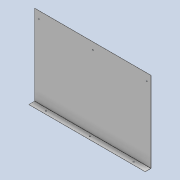
# Autodesk Inventor part: Tapa_interior_2
Saved by Autodesk Inventor 2021 (Build 250183000, 183)
## iProperties
Created: 2021-04-16
Part Number: Tapa_interior_2
Material: Genérico
Document SubType Name: Chapa
Designer: Admin
Density: 1 g/cm^3
Sheet Metal Rule: Por defecto_mm
Appearance: Valor por defecto
Flat Pattern Width: 36.1259 cm
Flat Pattern Length: 48.758 cm
Flat Pattern Area: 1761.43 cm^2
Sheet Metal Width: 361,259 mm
Sheet Metal Length: 487,580 mm
Sheet Metal Area: 176142,702 mm^2
Author: Admin
Autodesk Inventor part; units mm, degrees
ref_plane "YZ Plane" through (0, 0, 0) normal (1, 0, 0) x (0, 1, 0)
ref_plane "XZ Plane" through (0, 0, 0) normal (0, 1, 0) x (-1, 0, 0)
ref_plane "XY Plane" through (0, 0, 0) normal (0, 0, 1) x (1, 0, 0)
sketch "Boceto1" plane through (0, 0, 0) normal (0, 0, 1) x (1, 0, 0)
  line L0 (0, 0) -> (487.58, 0)
  line L1 (487.58, 0) -> (487.58, 337.58)
  line L2 (487.58, 337.58) -> (0, 337.58)
  line L3 (0, 337.58) -> (0, 0)
  dimension "d0" = 487.58
  dimension "d1" = 337.58
  measures "d0" distance of L2.end L1.end
  measures "d1" distance of L1.end L0.end
extrude "Placa1" add sketch "Boceto1" along normal blind 0.76
sketch "Boceto2" plane through (487.58, 0.76, 0) normal (0, -1, 0) x (1, 0, 0)
  line L0 (-487.58, 0) -> (0, 0)
  line L1 (0, 0) -> (0, 25)
  line L2 (0, 25) -> (-487.58, 25)
  line L3 (-487.58, 25) -> (-487.58, 0)
  constraints: 6 end point, 1 horizontal, 1 perpendicular, 1 vertical
edge flange "Pestaña1" height 25 angle 90 thickness 0.76 bend radius 0.76 thickness toward (0, -1, 0) relief straight relief width 0.76 relief depth 0.38 edges at (243.79, 0, 0.76) wall of the first edge with corners at (0, 0.76, 0) (487.58, 0.76, 0) (487.58, 0.76, 25) (0, 0.76, 25)
bend "Doblez1"
corner "Esquina1"
sketch "Boceto3" plane through (0, 0, 0) normal (0, 0, -1) x (-1, 0, 0)
  circle A0 centre (-469.48, 308.225) radius 2.5 projected
  circle A1 centre (-243.79, 308.225) radius 2.5 projected
  circle A2 centre (-18.1, 308.225) radius 2.5 projected
  point P0 (0, 0)
extrude "Cortar1" cut sketch "Boceto3" against normal blind 0.76
sketch "Boceto4" plane through (0, 0.76, 25) normal (0, 1, 0) x (1, 0, 0)
  line L0 (0, 23.48) -> (0, 0) projected
  line L1 (487.58, 23.48) -> (487.58, 0) projected
  line L2 (0, 0) -> (487.58, 0) projected
  line L3 (0, 23.48) -> (487.58, 23.48) projected
  line L4 (0, 23.48) -> (0, 0) projected
  circle A0 centre (60, 11.74) radius 2.5
  circle A1 centre (243.79, 11.74) radius 2.5
  circle A2 centre (427.58, 11.74) radius 2.5
  point P0 (0, 25)
  dimension "d15" = 60
  dimension "d16" = 60
  dimension "d17" = 5
  dimension "d18" = 5
  dimension "d19" = 5
  constraints: 3 centre point, 3 coincident
  measures "d15" distance from line of point (60, 11.74) L0
  measures "d16" distance from line of L1 point (427.58, 11.74)
  measures "d17" diameter of A0
  measures "d18" diameter of A1
  measures "d19" diameter of A2
extrude "Extrusión1" cut sketch "Boceto4" against normal through all contours A0 | A1 | A2
thread "Rosca1" size "M5x0.8" class "6H" standard "ANSI Metric M Profile" length 16
thread "Rosca2" size "M5x0.8" class "6H" standard "ANSI Metric M Profile" length 16
thread "Rosca3" size "M5x0.8" class "6H" standard "ANSI Metric M Profile" length 16
equation "\"d13\" = Grosor"
equation "\"d18\" = d17"
equation "\"d19\" = d17"
equation "\"d2\" = Grosor"
equation "\"d3\" = Anchura_desahogo_plegado"
equation "\"d4\" = Profundidad_desahogo_plegado"
equation "\"d5\" = Remanente_mínimo"
equation "\"d6\" = Radiodetransición"
equation "\"d9\" = Radio_pliegue"
equation "\"d10\" = Tamaño_destalonado"
equation "\"d11\" = TamañoSeparación"
equation "\"d12\" = Tamaño_de_radio_de_Jacobi"
equation "\"Radio_pliegue\" = Grosor"
equation "\"Anchura_desahogo_plegado\" = Grosor"
equation "\"Profundidad_desahogo_plegado\" = 0.5 * Grosor"
equation "\"Tamaño_destalonado\" = 4 * Grosor"
equation "\"Remanente_mínimo\" = 2 * Grosor"
equation "\"Radiodetransición\" = Radio_pliegue"
equation "\"Tamaño_de_radio_de_Jacobi\" = Radio_pliegue"
equation "\"TamañoSeparación\" = Grosor"
equation "\"Grosor\" = 0.76"
